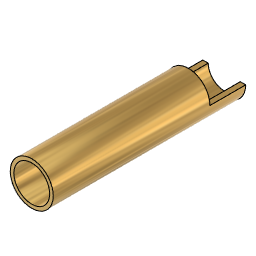
rigid phase connector jig (Autodesk Fusion 360 archive; units mm, degrees)
design "4mm bullet"
Autodesk Fusion 360 part; units mm, degrees
note: some values were not read from the file. Set by a fixed rule: which sketch regions a step uses.
imported_body "Base Feature1" makes body 1
sketch "Sketch1" plane through (0, -8, 0) normal (0, -1, 0) x (1, 0, 0)
  line L0 (-2.2173, 0.9184) -> (-2.3539, 0.4682) construction
  line L1 (-2.3539, 0.4682) -> (-2.4, 0) construction
  line L2 (-2.4, 0) -> (-2.3539, -0.4682) construction
  line L3 (-2.3539, -0.4682) -> (-2.2173, -0.9184) construction
  line L4 (-2.2173, -0.9184) -> (-1.9955, -1.3334) construction
  line L5 (-1.9955, -1.3334) -> (-1.6971, -1.6971) construction
  line L6 (-1.6971, -1.6971) -> (-1.3334, -1.9955) construction
  line L7 (-1.3334, -1.9955) -> (-0.9184, -2.2173) construction
  line L8 (-0.9184, -2.2173) -> (-0.4682, -2.3539) construction
  line L9 (-0.4682, -2.3539) -> (0, -2.4) construction
  line L10 (0, -2.4) -> (0.4682, -2.3539) construction
  line L11 (0.4682, -2.3539) -> (0.9184, -2.2173) construction
  line L12 (0.9184, -2.2173) -> (1.3334, -1.9955) construction
  line L13 (1.3334, -1.9955) -> (1.6971, -1.6971) construction
  line L14 (1.6971, -1.6971) -> (1.9955, -1.3334) construction
  line L15 (1.9955, -1.3334) -> (2.2173, -0.9184) construction
  line L16 (2.2173, -0.9184) -> (2.3539, -0.4682) construction
  line L17 (2.3539, -0.4682) -> (2.4, 0) construction
  line L18 (2.4, 0) -> (2.3539, 0.4682) construction
  line L19 (2.3539, 0.4682) -> (2.2173, 0.9184) construction
  line L20 (2.2173, 0.9184) -> (1.9955, 1.3334) construction
  line L21 (1.9955, 1.3334) -> (1.6971, 1.6971) construction
  line L22 (1.6971, 1.6971) -> (1.3334, 1.9955) construction
  line L23 (1.3334, 1.9955) -> (0.9184, 2.2173) construction
  line L24 (0.9184, 2.2173) -> (0.4682, 2.3539) construction
  line L25 (0.4682, 2.3539) -> (0, 2.4) construction
  line L26 (0, 2.4) -> (-0.4682, 2.3539) construction
  line L27 (-0.4682, 2.3539) -> (-0.9184, 2.2173) construction
  line L28 (-0.9184, 2.2173) -> (-1.3334, 1.9955) construction
  line L29 (-1.3334, 1.9955) -> (-1.6971, 1.6971) construction
  line L30 (-1.6971, 1.6971) -> (-1.9955, 1.3334) construction
  line L31 (-1.9955, 1.3334) -> (-2.2173, 0.9184) construction
  line L32 (-1.9616, -0.3902) -> (-2, 0) construction
  line L33 (-2, 0) -> (-1.9616, 0.3902) construction
  line L34 (-1.9616, 0.3902) -> (-1.8478, 0.7654) construction
  line L35 (-1.8478, 0.7654) -> (-1.6629, 1.1111) construction
  line L36 (-1.6629, 1.1111) -> (-1.4142, 1.4142) construction
  line L37 (-1.4142, 1.4142) -> (-1.1111, 1.6629) construction
  line L38 (-1.1111, 1.6629) -> (-0.7654, 1.8478) construction
  line L39 (-0.7654, 1.8478) -> (-0.3902, 1.9616) construction
  line L40 (-0.3902, 1.9616) -> (0, 2) construction
  line L41 (0, 2) -> (0.3902, 1.9616) construction
  line L42 (0.3902, 1.9616) -> (0.7654, 1.8478) construction
  line L43 (0.7654, 1.8478) -> (1.1111, 1.6629) construction
  line L44 (1.1111, 1.6629) -> (1.4142, 1.4142) construction
  line L45 (1.4142, 1.4142) -> (1.6629, 1.1111) construction
  line L46 (1.6629, 1.1111) -> (1.8478, 0.7654) construction
  line L47 (1.8478, 0.7654) -> (1.9616, 0.3902) construction
  line L48 (1.9616, 0.3902) -> (2, 0) construction
  line L49 (2, 0) -> (1.9616, -0.3902) construction
  line L50 (1.9616, -0.3902) -> (1.8478, -0.7654) construction
  line L51 (1.8478, -0.7654) -> (1.6629, -1.1111) construction
  line L52 (1.6629, -1.1111) -> (1.4142, -1.4142) construction
  line L53 (1.4142, -1.4142) -> (1.1111, -1.6629) construction
  line L54 (1.1111, -1.6629) -> (0.7654, -1.8478) construction
  line L55 (0.7654, -1.8478) -> (0.3902, -1.9616) construction
  line L56 (0.3902, -1.9616) -> (0, -2) construction
  line L57 (0, -2) -> (-0.3902, -1.9616) construction
  line L58 (-0.3902, -1.9616) -> (-0.7654, -1.8478) construction
  line L59 (-0.7654, -1.8478) -> (-1.1111, -1.6629) construction
  line L60 (-1.1111, -1.6629) -> (-1.4142, -1.4142) construction
  line L61 (-1.4142, -1.4142) -> (-1.6629, -1.1111) construction
  line L62 (-1.6629, -1.1111) -> (-1.8478, -0.7654) construction
  line L63 (-1.8478, -0.7654) -> (-1.9616, -0.3902) construction
  line L64 (0, 0) -> (-1.6629, -1.1111) construction
  circle A0 centre (0, 0) radius 2
  circle A1 centre (0, 0) radius 2.4
  constraint coincident L64.start A0.centre
  constraint coincident L61.end A0
  constraint concentric A0 A1
  constraint coincident L4.end A1
extrude "Extrude1" add sketch "Sketch1" against normal blind 17.5 separate body makes body 2
sketch "Sketch3" plane through (0, 9.5, 0) normal (0, 1, 0) x (-1, 0, 0)
  line L0 (-1.7917, -0.2361) -> (-1.7917, 0) construction
  line L1 (-1.7917, 0) -> (-2.389, 0) construction
  line L2 (-2.389, 0) -> (-2.3431, -0.4661) construction
  line L3 (-2.3431, -0.4661) -> (-2.2071, -0.9142) construction
  line L4 (-2.2071, -0.9142) -> (-1.9863, -1.3272) construction
  line L5 (-1.9863, -1.3272) -> (-1.6892, -1.6892) construction
  line L6 (-1.6892, -1.6892) -> (-1.3272, -1.9863) construction
  line L7 (-1.3272, -1.9863) -> (-0.9142, -2.2071) construction
  line L8 (-0.9142, -2.2071) -> (-0.4661, -2.3431) construction
  line L9 (-0.4661, -2.3431) -> (0, -2.389) construction
  line L10 (0, -2.389) -> (0.4661, -2.3431) construction
  line L11 (0.4661, -2.3431) -> (0.9142, -2.2071) construction
  line L12 (0.9142, -2.2071) -> (1.3272, -1.9863) construction
  line L13 (1.3272, -1.9863) -> (1.6892, -1.6892) construction
  line L14 (1.6892, -1.6892) -> (1.9863, -1.3272) construction
  line L15 (1.9863, -1.3272) -> (2.2071, -0.9142) construction
  line L16 (2.2071, -0.9142) -> (2.3431, -0.4661) construction
  line L17 (2.3431, -0.4661) -> (2.389, 0) construction
  line L18 (2.389, 0) -> (1.7917, 0) construction
  line L19 (1.7917, 0) -> (1.7573, -0.3495) construction
  line L20 (1.7573, -0.3495) -> (1.6553, -0.6857) construction
  line L21 (1.6553, -0.6857) -> (1.4898, -0.9954) construction
  line L22 (1.4898, -0.9954) -> (1.2669, -1.2669) construction
  line L23 (1.2669, -1.2669) -> (0.9954, -1.4898) construction
  line L24 (0.9954, -1.4898) -> (0.6857, -1.6553) construction
  line L25 (0.6857, -1.6553) -> (0.3495, -1.7573) construction
  line L26 (0.3495, -1.7573) -> (0, -1.7917) construction
  line L27 (0, -1.7917) -> (-0.3495, -1.7573) construction
  line L28 (-0.3495, -1.7573) -> (-0.6857, -1.6553) construction
  line L29 (-0.6857, -1.6553) -> (-0.9954, -1.4898) construction
  line L30 (-0.9954, -1.4898) -> (-1.2669, -1.2669) construction
  line L31 (-1.2669, -1.2669) -> (-1.4898, -0.9954) construction
  line L32 (-1.4898, -0.9954) -> (-1.6553, -0.6857) construction
  line L33 (-1.6553, -0.6857) -> (-1.7917, -0.2361) construction
  circle A0 centre (0, 0) radius 2
  circle A1 centre (0, 0) radius 2.4
  line L34 (-2.4, 0) -> (2.4, 0)
  circle A2 centre (0, 0) radius 1.7917
  constraint coincident A1 L34.start
  constraint coincident A1 L34.end
  constraint horizontal L34
  constraint collinear L1 L34
  constraint concentric A0 A2
  constraint coincident L0.end A2
extrude "Extrude2" add sketch "Sketch3" along normal blind 4 contours A0 A1 L34 | A0 L34 A2 picked at (2.2503, -0.2186) picked at (-1.9231, -0.0994) bodies 2
extrude "Extrude3" add sketch "Sketch3" against normal blind 2 contours A0 L34 A2 | A0 L34 A2 | L34 A2 | L34 A2 bodies 2
chamfer "Chamfer1" distance 2 angle 45 1 edges at (-1.8647, 7.5, 0.7232) on bodies 2
hidden bodies 1
named bodies: "Source"
